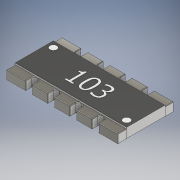
# Autodesk Inventor part: ResistorArray-3264
Saved by Autodesk Inventor 2018 (Build 220112000, 112)
## iProperties
Created: 2018-09-29
Part Number: ResistorArray-3264
Material: Copper
Document SubType Name: Modeling
Designer: Bradley
Density: 8.94 g/cm^3
Appearance: Smooth - White
Author: Bradley
Autodesk Inventor part; units mm, degrees
ref_plane "YZ Plane" through (0, 0, 0) normal (1, 0, 0) x (0, 1, 0)
ref_plane "XZ Plane" through (0, 0, 0) normal (0, 1, 0) x (-1, 0, 0)
ref_plane "XY Plane" through (0, 0, 0) normal (0, 0, 1) x (1, 0, 0)
sketch "Sketch1" plane through (0, 0, 0) normal (0, 0, 1) x (1, 0, 0)
  line L0 (-3.2, -1.1) -> (3.2, -1.1)
  line L1 (3.2, -1.1) -> (3.2, 1.1)
  line L2 (3.2, 1.1) -> (-3.2, 1.1)
  line L3 (-3.2, 1.1) -> (-3.2, -1.1)
  line L4 (-3.2, -1.1) -> (3.2, 1.1) construction
  line L5 (3.2, -1.1) -> (-3.2, 1.1) construction
  point P0 (0, 0)
  dimension "d0" = 6.4
  dimension "d1" = 2.2
  constraints: 12 end point, 2 midpoint, 2 parallel, 1 horizontal, 1 perpendicular
  measures "d0" distance of L2.end L1.end
  measures "d1" distance of L2.end L0.start
extrude "Extrusion1" add sketch "Sketch1" along normal mid plane 0.55
sketch "Sketch2" plane through (0, 0, 0) normal (0, 0, 1) x (1, 0, 0)
  line L0 (-3.2, -1.1) -> (3.2, -1.1) projected
  line L1 (3.2, -1.1) -> (3.2, 1.1) projected
  line L2 (3.2, 1.1) -> (-3.2, 1.1) projected
  line L3 (-3.2, 1.1) -> (-3.2, -1.1) projected
  line L4 (3.2, 1.1) -> (-3.2, 1.1) projected
  line L5 (-3.19, 1.1) -> (-2.09, 1.1)
  line L6 (-2.09, 1.1) -> (-2.09, 1.6)
  line L7 (-2.09, 1.6) -> (-3.19, 1.6)
  line L8 (-3.19, 1.6) -> (-3.19, 1.1)
  line L9 (-3.19, -1.1) -> (-2.09, -1.1)
  line L10 (-2.09, -1.1) -> (-2.09, -1.6)
  line L11 (-2.09, -1.6) -> (-3.19, -1.6)
  line L12 (-3.19, -1.6) -> (-3.19, -1.1)
  line L13 (3.19, -1.1) -> (2.09, -1.1)
  line L14 (2.09, -1.1) -> (2.09, -1.6)
  line L15 (2.09, -1.6) -> (3.19, -1.6)
  line L16 (3.19, -1.6) -> (3.19, -1.1)
  line L17 (3.19, 1.1) -> (2.09, 1.1)
  line L18 (2.09, 1.1) -> (2.09, 1.6)
  line L19 (2.09, 1.6) -> (3.19, 1.6)
  line L20 (3.19, 1.6) -> (3.19, 1.1)
  line L21 (-1.72, 1.1) -> (-0.82, 1.1)
  line L22 (-0.82, 1.1) -> (-0.82, 1.6)
  line L23 (-0.82, 1.6) -> (-1.72, 1.6)
  line L24 (-1.72, 1.6) -> (-1.72, 1.1)
  line L25 (-3.2, -1.1) -> (3.2, -1.1) projected
  line L26 (-1.72, -1.1) -> (-0.82, -1.1)
  line L27 (-0.82, -1.1) -> (-0.82, -1.6)
  line L28 (-0.82, -1.6) -> (-1.72, -1.6)
  line L29 (-1.72, -1.6) -> (-1.72, -1.1)
  line L30 (-0.45, -1.1) -> (0.45, -1.1)
  line L31 (0.45, -1.1) -> (0.45, -1.6)
  line L32 (0.45, -1.6) -> (-0.45, -1.6)
  line L33 (-0.45, -1.6) -> (-0.45, -1.1)
  line L34 (0.45, 1.6) -> (-0.45, 1.6)
  line L35 (-0.45, 1.6) -> (-0.45, 1.1)
  line L36 (0.45, 1.1) -> (0.45, 1.6)
  line L37 (-0.45, 1.1) -> (0.45, 1.1)
  line L38 (0.82, -1.1) -> (1.72, -1.1)
  line L39 (1.72, -1.1) -> (1.72, -1.6)
  line L40 (1.72, -1.6) -> (0.82, -1.6)
  line L41 (0.82, -1.6) -> (0.82, -1.1)
  line L42 (1.72, 1.6) -> (0.82, 1.6)
  line L43 (0.82, 1.6) -> (0.82, 1.1)
  line L44 (1.72, 1.1) -> (1.72, 1.6)
  line L45 (0.82, 1.1) -> (1.72, 1.1)
  point P0 (0, 0)
  point P1 (0, 1.1)
  dimension "d4" = 1.1
  dimension "d5" = 0.9
  dimension "d6" = 3.2
  dimension "d9" = 1.27
  dimension "d18" = 0.01
  dimension "d19" = 0.01
  constraints: 80 end point, 14 point on line, 12 parallel, 7 horizontal, 6 perpendicular, 5 collinear, 4 equal length, 2 midpoint, 31 other
  measures "d4" distance of L6.end L7.end
  measures "d5" distance of L22.end L23.end
  measures "d6" distance between parallel lines of L11 L7
  measures "d9" distance of L26.end L30.end
  measures "d18" distance between parallel lines of L1 L20
  measures "d19" distance between parallel lines of L3 L8
extrude "Extrusion2" add sketch "Sketch2" along normal blind 0.2 and the other way blind 0.325 contours L0 L10 L11 L12 | L8 L7 L6 L2 | L0 L27 L28 L29 | L24 L23 L22 L2 | L0 L31 L32 L33 | L35 L34 L36 L2 | L0 L39 L40 L41 | L43 L42 L44 L2 | L0 L16 L15 L14 | L18 L19 L20 L2
sketch "Sketch3" plane through (0, 0, 0.275) normal (0, 0, 1) x (1, 0, 0)
  circle A0 centre (-2.85, 0.75) radius 0.2
  circle A1 centre (2.85, -0.75) radius 0.2
  line L0 (-3.2, -1.1) -> (3.2, -1.1) projected
  line L1 (3.2, -1.1) -> (3.2, 1.1) projected
  line L2 (3.2, 1.1) -> (-3.2, 1.1) projected
  line L3 (-3.2, 1.1) -> (-3.2, -1.1) projected
  circle A2 centre (-2.85, 0.75) radius 0.35 construction
  circle A3 centre (2.85, -0.75) radius 0.35 construction
  point P0 (0, 0)
  dimension "d20" = 0.4
  dimension "d21" = 0.7
  constraints: 4 centre point, 4 tangent, 2 coincident, 2 equal radius
  measures "d20" diameter of A0
  measures "d21" diameter of A2
extrude "Extrusion3" add sketch "Sketch3" along normal blind 0.01 contours A0 | A1
fillet "Fillet3" radius 0.18 16 edges at (-2.09, -1.1, -0.0375) (-1.72, -1.1, -0.0375) (-0.82, -1.1, -0.0375) (-0.45, -1.1, -0.0375) (0.45, -1.1, -0.0375) (0.82, -1.1, -0.0375) (1.72, -1.1, -0.0375) (2.09, -1.1, -0.0375) (2.09, 1.1, -0.0375) (1.72, 1.1, -0.0375) (0.82, 1.1, -0.0375) (0.45, 1.1, -0.0375) (-0.45, 1.1, -0.0375) (-0.82, 1.1, -0.0375) (-1.72, 1.1, -0.0375) (-2.09, 1.1, -0.0375)
fillet "Fillet1" radius 0.03 110 edges at (-2.09, -1.35, -0.325) (-2.64, -1.6, -0.325) (-3.19, -1.35, -0.325) (-2.64, -1.1, -0.325) (-2.09, -1.6, -0.0625) (-2.64, -1.6, 0.2) (-3.19, -1.6, -0.0625) (-3.19, -1.35, 0.2) (-3.19, -1.1, -0.3) (-2.09, -1.1, -0.3) (-2.09, -1.44, 0.2) (-2.64, 1.1, -0.325) (-3.19, 1.35, -0.325) (-2.64, 1.6, -0.325) (-2.09, 1.35, -0.325) (-3.19, 1.35, 0.2) (-3.19, 1.6, -0.0625) (-3.19, 1.1, -0.3) (-2.64, 1.6, 0.2) (-2.09, 1.6, -0.0625) (-2.09, 1.44, 0.2) (-2.09, 1.1, -0.3) (1.27, -1.1, -0.325) (1.72, -1.35, -0.325) (1.27, -1.6, -0.325) (0.82, -1.35, -0.325) (1.72, -1.44, 0.2) (1.72, -1.6, -0.0625) (1.72, -1.1, -0.3) (1.27, -1.6, 0.2) (0.82, -1.6, -0.0625) (0.82, -1.44, 0.2) (0.82, -1.1, -0.3) (-1.27, 1.1, -0.325) (-1.72, 1.35, -0.325) (-1.27, 1.6, -0.325) (-0.82, 1.35, -0.325) (-1.72, 1.44, 0.2) (-1.72, 1.6, -0.0625) (-1.72, 1.1, -0.3) (-1.27, 1.6, 0.2) (-0.82, 1.6, -0.0625) (-0.82, 1.44, 0.2) (-0.82, 1.1, -0.3) (-0.82, -1.1, -0.3) (-1.27, -1.1, -0.325) (-1.72, -1.1, -0.3) (-1.72, -1.35, -0.325) (-0.82, -1.35, -0.325) (-1.27, -1.6, -0.325) (-0.82, -1.44, 0.2) (-0.82, -1.6, -0.0625) (-1.27, -1.6, 0.2) (-1.72, -1.6, -0.0625) (-1.72, -1.44, 0.2) (0, 1.1, -0.325) (-0.45, 1.35, -0.325) (0, 1.6, -0.325) (0.45, 1.35, -0.325) (-0.45, 1.1, -0.3) (-0.45, 1.44, 0.2) (-0.45, 1.6, -0.0625) (0, 1.6, 0.2) (0.45, 1.6, -0.0625) (0.45, 1.44, 0.2) (0.45, 1.1, -0.3) (0, -1.1, -0.325) (0.45, -1.35, -0.325) (0, -1.6, -0.325) (-0.45, -1.35, -0.325) (0.45, -1.44, 0.2) (0.45, -1.6, -0.0625) (0.45, -1.1, -0.3) (0, -1.6, 0.2) (-0.45, -1.6, -0.0625) (-0.45, -1.44, 0.2) (-0.45, -1.1, -0.3) (1.27, 1.1, -0.325) (0.82, 1.35, -0.325) (1.27, 1.6, -0.325) (1.72, 1.35, -0.325) (0.82, 1.44, 0.2) (0.82, 1.6, -0.0625) (0.82, 1.1, -0.3) (1.27, 1.6, 0.2) (1.72, 1.6, -0.0625) (1.72, 1.44, 0.2) (1.72, 1.1, -0.3) (2.09, 1.1, -0.3) (2.64, 1.1, -0.325) (3.19, 1.1, -0.3) (3.19, 1.35, -0.325) (2.09, 1.35, -0.325) (2.64, 1.6, -0.325) (2.09, 1.44, 0.2) (2.09, 1.6, -0.0625) (2.64, 1.6, 0.2) (3.19, 1.6, -0.0625) (3.19, 1.35, 0.2) (3.19, -1.1, -0.3) (2.64, -1.1, -0.325) (2.09, -1.1, -0.3) (2.09, -1.35, -0.325) (3.19, -1.35, -0.325) (2.64, -1.6, -0.325) (3.19, -1.35, 0.2) (3.19, -1.6, -0.0625) (2.64, -1.6, 0.2) (2.09, -1.6, -0.0625) (2.09, -1.44, 0.2)
sketch "Sketch4" plane through (0, 0, 0.275) normal (0, 0, 1) x (1, 0, 0)
  line L0 (-3.2, 1.1) -> (-3.2, -1.1) construction
  line L1 (-3.2, 0) -> (3.1936, 0) construction
  line L2 (-0.4894, -0.5) -> (-0.9773, -0.5)
  line L3 (-0.9773, -0.5) -> (-0.9773, -0.3979)
  line L4 (-0.9773, -0.3979) -> (-0.7957, -0.3979)
  line L5 (-0.7957, -0.3979) -> (-0.7957, 0.2723)
  line L6 (-0.7957, 0.2723) -> (-0.9773, 0.2723)
  line L7 (-0.9773, 0.2723) -> (-0.9773, 0.3639)
  spline S0 degree 2 poles (-0.9773, 0.3639) (-0.8743, 0.3639) (-0.7771, 0.4222) (-0.7706, 0.5032) knots 0 0 0 1 2 2 2
  line L8 (-0.7706, 0.5032) -> (-0.6669, 0.5032)
  line L9 (-0.6669, 0.5032) -> (-0.6669, -0.3979)
  line L10 (-0.6669, -0.3979) -> (-0.4894, -0.3979)
  line L11 (-0.4894, -0.3979) -> (-0.4894, -0.5)
  spline S1 degree 2 poles (0.3169, 0) (0.3169, -0.269) (0.1605, -0.5211) (-0.0024, -0.5211) knots 0 0 0 1 2 2 2
  spline S2 degree 2 poles (-0.0024, -0.5211) (-0.1677, -0.5211) (-0.3225, -0.2642) (-0.3225, -0.0008) knots 0 0 0 1 2 2 2
  spline S3 degree 2 poles (-0.3225, -0.0008) (-0.3225, 0.2699) (-0.1661, 0.5203) (-0.0024, 0.5203) knots 0 0 0 1 2 2 2
  spline S4 degree 2 poles (-0.0024, 0.5203) (0.1621, 0.5203) (0.3169, 0.2609) (0.3169, 0) knots 0 0 0 1 2 2 2
  spline S5 degree 2 poles (0.1451, -0.3047) (0.1646, -0.2553) (0.1808, -0.1029) (0.1808, 0) knots 0 0 0 1 2 2 2
  spline S6 degree 2 poles (0.1808, 0) (0.1808, 0.1029) (0.1646, 0.2545) (0.1443, 0.3055) knots 0 0 0 1 2 2 2
  spline S7 degree 2 poles (0.1443, 0.3055) (0.124, 0.3566) (0.0535, 0.4092) (-0.0024, 0.4092) knots 0 0 0 1 2 2 2
  spline S8 degree 2 poles (-0.0024, 0.4092) (-0.0583, 0.4092) (-0.1304, 0.3566) (-0.1515, 0.3039) knots 0 0 0 1 2 2 2
  spline S9 degree 2 poles (-0.1515, 0.3039) (-0.1717, 0.2528) (-0.1863, 0.0972) (-0.1863, -0.0008) knots 0 0 0 1 2 2 2
  spline S10 degree 2 poles (-0.1863, -0.0008) (-0.1863, -0.1062) (-0.1734, -0.2472) (-0.1523, -0.3023) knots 0 0 0 1 2 2 2
  spline S11 degree 2 poles (-0.1523, -0.3023) (-0.1329, -0.3541) (-0.0607, -0.41) (-0.0024, -0.41) knots 0 0 0 1 2 2 2
  spline S12 degree 2 poles (-0.0024, -0.41) (0.0527, -0.41) (0.1248, -0.3574) (0.1451, -0.3047) knots 0 0 0 1 2 2 2
  spline S13 degree 2 poles (0.7148, 0.4052) (0.6783, 0.4052) (0.6062, 0.3874) (0.5714, 0.3736) knots 0 0 0 1 2 2 2
  spline S14 degree 2 poles (0.5714, 0.3736) (0.5389, 0.3598) (0.4911, 0.3306) (0.4725, 0.3177) knots 0 0 0 1 2 2 2
  line L12 (0.4725, 0.3177) -> (0.4644, 0.3177)
  line L13 (0.4644, 0.3177) -> (0.4644, 0.4595)
  spline S15 degree 2 poles (0.4644, 0.4595) (0.5082, 0.483) (0.6581, 0.5211) (0.7253, 0.5211) knots 0 0 0 1 2 2 2
  spline S16 degree 2 poles (0.7253, 0.5211) (0.7934, 0.5211) (0.8947, 0.4935) (0.936, 0.4643) knots 0 0 0 1 2 2 2
  spline S17 degree 2 poles (0.936, 0.4643) (0.9798, 0.4327) (1.0252, 0.3412) (1.0252, 0.2796) knots 0 0 0 1 2 2 2
  spline S18 degree 2 poles (1.0252, 0.2796) (1.0252, 0.1969) (0.9166, 0.0721) (0.8404, 0.0559) knots 0 0 0 1 2 2 2
  line L14 (0.8404, 0.0559) -> (0.8404, 0.0462)
  spline S19 degree 2 poles (0.8404, 0.0462) (0.872, 0.0397) (0.9441, 0.0105) (0.9749, -0.0186) knots 0 0 0 1 2 2 2
  spline S20 degree 2 poles (0.9749, -0.0186) (1.0057, -0.047) (1.0446, -0.1378) (1.0446, -0.2034) knots 0 0 0 1 2 2 2
  spline S21 degree 2 poles (1.0446, -0.2034) (1.0446, -0.2707) (0.9984, -0.3849) (0.9563, -0.4287) knots 0 0 0 1 2 2 2
  spline S22 degree 2 poles (0.9563, -0.4287) (0.9125, -0.4741) (0.7885, -0.5211) (0.7099, -0.5211) knots 0 0 0 1 2 2 2
  spline S23 degree 2 poles (0.7099, -0.5211) (0.6346, -0.5211) (0.4871, -0.4846) (0.4368, -0.4595) knots 0 0 0 1 2 2 2
  line L15 (0.4368, -0.4595) -> (0.4368, -0.3177)
  line L16 (0.4368, -0.3177) -> (0.4466, -0.3177)
  spline S24 degree 2 poles (0.4466, -0.3177) (0.4887, -0.3485) (0.6313, -0.4052) (0.7018, -0.4052) knots 0 0 0 1 2 2 2
  spline S25 degree 2 poles (0.7018, -0.4052) (0.7432, -0.4052) (0.8258, -0.3793) (0.8534, -0.3493) knots 0 0 0 1 2 2 2
  spline S26 degree 2 poles (0.8534, -0.3493) (0.8801, -0.3193) (0.9085, -0.248) (0.9085, -0.1937) knots 0 0 0 1 2 2 2
  spline S27 degree 2 poles (0.9085, -0.1937) (0.9085, -0.1394) (0.8769, -0.0689) (0.8485, -0.0486) knots 0 0 0 1 2 2 2
  spline S28 degree 2 poles (0.8485, -0.0486) (0.8201, -0.0284) (0.7432, -0.013) (0.6978, -0.013) knots 0 0 0 1 2 2 2
  line L17 (0.6978, -0.013) -> (0.6411, -0.013)
  line L18 (0.6411, -0.013) -> (0.6411, 0.0981)
  line L19 (0.6411, 0.0981) -> (0.6856, 0.0981)
  spline S29 degree 2 poles (0.6856, 0.0981) (0.7756, 0.0981) (0.889, 0.184) (0.889, 0.2658) knots 0 0 0 1 2 2 2
  spline S30 degree 2 poles (0.889, 0.2658) (0.889, 0.3039) (0.8599, 0.3582) (0.8364, 0.3744) knots 0 0 0 1 2 2 2
  spline S31 degree 2 poles (0.8364, 0.3744) (0.8112, 0.3914) (0.7496, 0.4052) (0.7148, 0.4052) knots 0 0 0 1 2 2 2
  point P0 (0, 0)
  constraints: 2 end point, 2 horizontal, 1 midpoint
extrude "Extrusion4" add sketch "Sketch4" along normal blind 0.01
equation "\"d19\" = d18"
body "Solid1"
